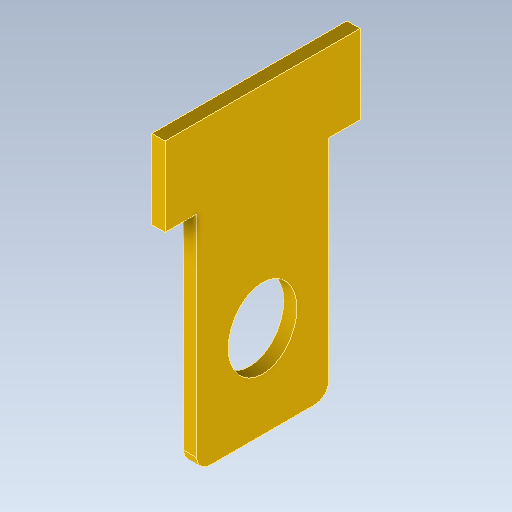
# Autodesk Inventor part: 555_Terminal
Saved by Autodesk Inventor 2021 (Build 250183000, 183)
## iProperties
Created: 2021-08-07
Part Number: 555_Terminal
Material: 銅
Document SubType Name: Modeling
Designer: Hagihara Yuya
Density: 8.94 g/cm^3
Appearance: ゴールド
Author: Hagihara Yuya
Autodesk Inventor part; units mm, degrees
ref_plane "YZ Plane" through (0, 0, 0) normal (1, 0, 0) x (0, 1, 0)
ref_plane "XZ Plane" through (0, 0, 0) normal (0, 1, 0) x (-1, 0, 0)
ref_plane "XY Plane" through (0, 0, 0) normal (0, 0, 1) x (1, 0, 0)
sketch "スケッチ1" plane through (0, 0, 0) normal (1, 0, 0) x (0, 1, 0)
  line L0 (3.7, 0) -> (-3.7, 0)
  line L1 (-3.7, 0) -> (-3.7, -3)
  line L2 (-3.7, -3) -> (3.7, -3)
  line L3 (3.7, -3) -> (3.7, 0)
  line L4 (2.5, -3) -> (-2.5, -3)
  line L5 (-2.5, -3) -> (-2.5, -11.5)
  line L6 (-2.5, -11.5) -> (2.5, -11.5)
  line L7 (2.5, -11.5) -> (2.5, -3)
  point P0 (0, 0)
  point P1 (0, 0)
  point P2 (0, -3)
  dimension "d0" = 7.4
  dimension "d1" = 3
  dimension "d2" = 5
  dimension "d3" = 8.5
  constraints: 16 end point, 4 parallel, 3 midpoint, 2 horizontal, 2 perpendicular, 1 coincident, 1 point on line
  measures "d0" distance of L0.start L0.end
  measures "d1" distance of L0.end L1.end
  measures "d2" distance of L5.end L6.end
  measures "d3" distance of L4.end L5.end
extrude "押し出し1" add sketch "スケッチ1" along normal blind 0.5
sketch "スケッチ2" plane through (0.5, 0, 0) normal (1, 0, 0) x (0, 0, -1)
  ellipse E0 centre (8, 0) end of major axis (9.5, 0) minor radius 1.3
  line L0 (0, 3.7) -> (0, -3.7) projected
  line L1 (11.5, -2.5) -> (11.5, 2.5) projected
  point P0 (0, 0)
  point P1 (0, 0)
  dimension "d6" = 1.3
  dimension "d7" = 1.5
  dimension "d8" = 3.5
  constraints: 1 centre point, 1 horizontal alignment, 1 midpoint, 1 other
  measures "d8" distance from line of L1 E0.centre
extrude "押し出し2" cut sketch "スケッチ2" against normal through all
fillet "フィレット1" radius 0.5 2 edges at (0.25, -2.5, -11.5) (0.25, 2.5, -11.5)
